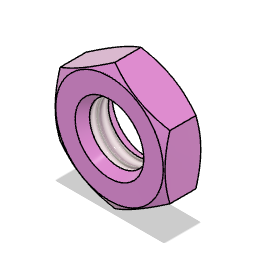
stepper_with_joints v8 (Autodesk Fusion 360 archive; units mm, degrees)
design "Hexagon Thin Nut DIN 439-2 - M5 x 0.8 Steel 6 Plain"
description: Hexagon Thin Nut DIN 439-2 - M5 x 0.8
Autodesk Fusion 360 part; units mm, degrees
note: some values were not read from the file. Chosen so that the rebuilt part matches the saved one: that a step has no effect; which face or edge a step refers to; how an offset face is resized. Set by a fixed rule: which sketch regions a step uses.
sketch "Sketch1" plane through (0, 0, 0) normal (0, 1, 0) x (1, 0, 0)
  line L0 (0, 0) -> (0, -2.7)
  line L1 (-2.5, 0) -> (-3.92, 0)
  line L2 (-3.92, 0) -> (-4.62, -0.4041)
  line L3 (-4.62, -0.4041) -> (-4.62, -2.2959)
  line L4 (-4.62, -2.2959) -> (-3.92, -2.7)
  line L5 (-3.92, -2.7) -> (-2.5, -2.7)
  line L6 (-2.5, -2.7) -> (-2.5, 0)
  dimension "d121" = 5
  dimension "d122" = 30
  dimension "d123" = 30
  dimension "d126" = 2.7
  dimension "d128" = 9.24
  dimension "d172" = 7.84
  constraint vertical L0
  constraint coincident L0 L0.end
  constraint coincident origin L0
  constraint horizontal L1
  constraint perpendicular L1 L3
  constraint perpendicular L3 L5
  constraint perpendicular L5 L6
  constraint coincident L0.start L1
  constraint coincident L0.start origin
  constraint coincident L0.end L5
  constraint equal L1 L5
  measures "d122" angle of L1 L2
  measures "d123" angle of L4 L5
  measures "d126" distance of L1.start L5.end
revolve "Revolve1" add sketch "Sketch1" angle 360 about axis through (0, 0, 0) along (0, 0, 1)
sketch "Sketch8" plane through (0, 0, 2.7) normal (0, 0, 1) x (1, 0, 0)
  line L0 (0, 0) -> (-8, 0) construction
  line L1 (-4, -2.3118) -> (-4, 2.3118)
  circle A0 centre (0, 0) radius 2.5
  circle A1 centre (0, 0) radius 4.62
  dimension "d114" = 4
  constraint horizontal L0
  constraint perpendicular L0 L1
  constraint midpoint L0 L1
  constraint coincident L0.start A0.centre
  constraint coincident L1.end A1
  measures "d114" distance of L0.start L1
extrude "Extrude5" cut sketch "Sketch8" against normal blind 2.7 contours L1 A1 picked at (-4.1, -0.5631)
pattern_circular "C-Pattern2" count 6 over 360 about axis through (0, 0, 1.75) along (0, 0, 1) of "Extrude5"
thread "Thread3" "ISO Metric profile 5.0 M5x0.8 6H" major diameter 5.12 minor diameter 4.234 pitch 0.8 angle 60 resizes the face on face at (-2.4969, 0.1246, 1.8)
sketch "Sketch12" plane through (0, 0, 0) normal (0, 1, 0) x (1, 0, 0)
  line L0 (2.117, -2.7) -> (-2.117, -2.7)
  line L1 (3.92, -2.7) -> (-3.92, -2.7)
  line L2 (3.92, 0) -> (-3.92, 0)
  line L3 (2.117, 0) -> (-2.117, 0)
  line L4 (-2.5, 0) -> (0, 0)
  line L5 (-1.7206, -1.35) -> (-2.5, 0)
  line L6 (-2.5, -2.7) -> (0, -2.7)
  line L7 (-1.7206, -1.35) -> (-2.5, -2.7)
  line L8 (0, 0) -> (0, -2.7)
  dimension "d165" = 60
  dimension "d169" = 60
  dimension "d170" = 2.5
  constraint horizontal L4
  constraint collinear L1 L6
  constraint coincident L5.start L7.start
  constraint vertical L4.start L6.start
  constraint coincident L1 L6.end
  constraint coincident L6.end L8.end
  constraint coincident L4.end L8.start
  measures "d165" angle of L2 L5
  measures "d169" angle of L6 L7
  measures "d170" distance of L4.start L4.end
revolve "Revolve3" cut sketch "Sketch12" angle 360 about axis through (0, 0, 1.75) along (0, 0, 1)
equation "adsk_nheig = 2.70 mm"
equation "adsk_maxdia = 9.24 mm"
equation "adsk_nomdia = 5.00 mm"
equation "d89 = -adsk_nheig"
equation "adsk_waflat = 8.00 mm"
equation "d114 = adsk_waflat / 2"
equation "adsk_chamang1 = 30.00 deg"
equation "adsk_chamang2 = 30.00 deg"
equation "d121 = adsk_nomdia"
equation "d122 = adsk_chamang1"
equation "d123 = adsk_chamang2"
equation "d126 = adsk_nheig"
equation "d128 = adsk_maxdia"
equation "d163 = adsk_nheig"
equation "d170 = adsk_nomdia * 0.5"
equation "adsk_beardia = adsk_waflat * 0.98"
equation "d172 = adsk_beardia"

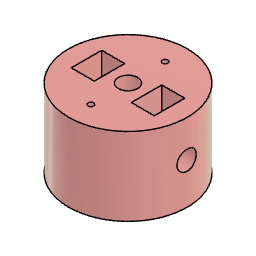
design "nema17 shaft coupler"
Autodesk Fusion 360 part; units mm, degrees
sketch "Sketch1" plane through (0, 0, 0) normal (0, 0, 1) x (1, 0, 0)
  circle A0 centre (0, 0) radius 21
  circle A1 centre (0, 0) radius 2.6
  dimension "d1" = 42
  dimension "d2" = 5.2
  constraint coincident A0.centre A1.centre
  measures "d1" diameter of A0
  measures "d2" diameter of A1
extrude "Extrude1" [suppressed]
sketch "Sketch2" plane through (0, 0, 15) normal (0, 0, 1) x (-1, 0, 0)
  circle A0 centre (0, 0) radius 1.375
  circle A1 centre (0, 0) radius 21
  line L0 (-5, -5.1) -> (-10.2, -5.1)
  line L1 (-10.2, -5.1) -> (-10.2, 5.1)
  line L2 (-10.2, 5.1) -> (-5, 5.1)
  line L3 (-5, 5.1) -> (-5, -5.1)
  line L4 (0, 0) -> (-5, 0)
  dimension "d5" = 5.2
  dimension "d6" = 10.2
  dimension "d7" = 5
  constraint horizontal L0
  constraint vertical L1
  constraint horizontal L2
  constraint vertical L3
  constraint coincident A0.centre A1.centre
  constraint horizontal L4
  constraint midpoint L3 L4.end
  measures "d5" distance of L0.start L0.end
  measures "d6" distance of L0.start L2.end
  measures "d7" distance of A0.centre L4.end
extrude "Extrude2" cut sketch "Sketch2" against normal blind 10 contours L0 L1 L2 L3
ref_plane "WorkPlane1" through (0, 0, 22) normal (0, 0, 1) x (1, 0, 0)
sketch "Sketch3" plane through (5, 0, 0) normal (1, 0, 0) x (0, 1, 0)
  line L0 (5.1, 15) -> (-5.1, 15)
  line L1 (-5.1, 15) -> (-5.1, 5)
  line L2 (-5.1, 5) -> (5.1, 5)
  line L3 (5.1, 5) -> (5.1, 15)
  circle A0 centre (0, 5) radius 3.1
  dimension "d11" = 6.2
  constraint midpoint L2 A0.centre
  measures "d11" diameter of A0
extrude "Extrude3" [no effect]
sketch "Sketch4" plane through (0, 0, 0) normal (0, 0, 1) x (1, 0, 0)
  circle A0 centre (0, 0) radius 16
  circle A1 centre (0, 0) radius 2.6
  dimension "d15" = 32
  dimension "d16" = 5.2
  constraint coincident A0.centre A1.centre
  measures "d15" diameter of A0
  measures "d16" diameter of A1
extrude "Extrude4" add sketch "Sketch4" along normal blind 21 separate body
sketch "Sketch5" plane through (0, 0, 21) normal (0, 0, 1) x (-1, 0, 0)
  circle A0 centre (0, 0) radius 2.6
  circle A1 centre (0, 0) radius 16
  line L0 (-5, -4.1) -> (-11.2, -4.1)
  line L1 (-11.2, -4.1) -> (-11.2, 4.1)
  line L2 (-11.2, 4.1) -> (-5, 4.1)
  line L3 (-5, 4.1) -> (-5, -4.1)
  line L4 (0, 0) -> (-5, 0) construction
  dimension "d19" = 6.2
  dimension "d20" = 8.2
  dimension "d21" = 5
  constraint horizontal L0
  constraint vertical L1
  constraint horizontal L2
  constraint vertical L3
  constraint coincident A0.centre A1.centre
  constraint horizontal L4
  constraint midpoint L3 L4.end
  measures "d19" distance of L0.start L0.end
  measures "d20" distance of L0.start L2.end
  measures "d21" distance of A0.centre L4.end
extrude "Extrude5" cut sketch "Sketch5" against normal blind 10 contours L0 L1 L2 L3
sketch "Sketch6" plane through (5, 0, 0) normal (1, 0, 0) x (0, 1, 0)
  line L0 (4.1, 21) -> (-4.1, 21)
  line L1 (-4.1, 21) -> (-4.1, 11)
  line L2 (-4.1, 11) -> (4.1, 11)
  line L3 (4.1, 11) -> (4.1, 21)
  circle A0 centre (0, 11) radius 2.6
  dimension "d24" = 5.2
  constraint midpoint L2 A0.centre
  measures "d24" diameter of A0
extrude "Extrude6" cut sketch "Sketch6" along normal through all and the other way blind 5 contours L2 A0 | L2 A0
sketch "Sketch7" plane through (5, 0, 0) normal (1, 0, 0) x (0, 1, 0)
  arc A0 (2.6, 11) -> (-2.6, 11) centre (0, 11) ccw
  line L0 (2.6, 11) -> (4.1, 11)
  line L1 (4.1, 11) -> (4.1, 21)
  line L2 (4.1, 21) -> (-4.1, 21)
  line L3 (-4.1, 21) -> (-4.1, 11)
  line L4 (-4.1, 11) -> (-2.6, 11)
  line L5 (4.1, 13.3671) -> (0, 15.7343)
  line L6 (0, 15.7343) -> (-4.1, 13.3671)
  line L7 (-4.1, 13.3671) -> (-4.1, 8.6329)
  line L8 (-4.1, 8.6329) -> (0, 6.2657)
  line L9 (0, 6.2657) -> (4.1, 8.6329)
  line L10 (4.1, 8.6329) -> (4.1, 13.3671)
  point P0 (0, 11)
  constraint coincident P0 A0.centre
  constraint midpoint L0.end L10
extrude "Extrude7" cut sketch "Sketch7" along normal blind 5.2 contours A0 L0 L4 L7 L8 L9 L10 | A0 L0 L1 L3 L4 L5 L6 L7 L10
sketch "Sketch8" plane through (0, 0, 21) normal (0, 0, 1) x (-1, 0, 0)
  line L0 (-11.2, -4.1) -> (-11.2, 4.1)
  line L1 (-11.2, 4.1) -> (-5, 4.1)
  line L2 (-5, 4.1) -> (-5, -4.1)
  line L3 (-5, -4.1) -> (-11.2, -4.1)
  circle A0 centre (0, 0) radius 2.6
  circle A1 centre (0, 0) radius 16
  circle A2 centre (0, -10) radius 0.75
  line L4 (0, 0) -> (16, 0) construction
  circle A3 centre (0, 10) radius 0.75
  dimension "d30" = 1.5
  dimension "d31" = 10
  constraint coincident A0.centre A1.centre
  constraint coincident A1 L4.end
  constraint horizontal L4
  constraint vertical A0.centre A2.centre
  constraint symmetric A2 L4 A3
  measures "d30" diameter of A2
  measures "d31" vertical distance of A0.centre A2.centre
extrude "Extrude8" cut sketch "Sketch8" against normal blind 6 contours A2 | A3
mirror "Mirror1" about plane through (0, 0, 0) normal (1, 0, 0) of "Extrude5", "Extrude6", "Extrude7"

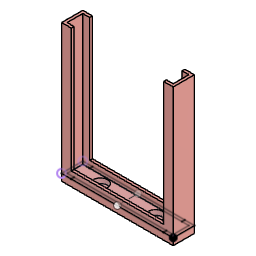
design "pan holder 2"
Autodesk Fusion 360 part; units mm, degrees
sketch "Sketch1" plane through (0, 0, 0) normal (0, 0, 1) x (1, 0, 0)
  line L0 (0, 0) -> (81.3, 0)
  line L1 (81.3, 0) -> (81.3, 15.4)
  line L2 (81.3, 15.4) -> (0, 15.4)
  line L3 (0, 15.4) -> (0, 0)
  dimension "d8" = 81.3
  dimension "d9" = 15.4
  constraint horizontal L0
  constraint vertical L1
  constraint horizontal L2
  constraint vertical L3
  constraint coincident L0.start L3.end
  measures "d8" distance of L0.start L0.end
  measures "d9" distance of L0.start L2.end
extrude "Extrude1" add sketch "Sketch1" along normal blind 5
sketch "Sketch2" plane through (0, 0, 5) normal (0, 0, 1) x (-1, 0, 0)
  line L0 (0, -15.4) -> (0, 0)
  line L1 (0, 0) -> (-81.3, 0)
  line L2 (-81.3, 0) -> (-81.3, -15.4)
  line L3 (-81.3, -15.4) -> (0, -15.4)
  circle A0 centre (-20.65, -7.7) radius 2.6
  circle A1 centre (-20.65, -7.7) radius 5.1
  line L4 (-40.65, -15.4) -> (-40.65, -7.6842) construction
  line L5 (-40.65, -7.7) -> (-81.3, -7.7) construction
  circle A2 centre (-60.65, -7.7) radius 5.1
  circle A3 centre (-60.65, -7.7) radius 2.6
  dimension "d16" = 5.2
  dimension "d18" = 7.7
  dimension "d19" = 10.2
  dimension "d34" = 20
  constraint midpoint L3 L4.start
  constraint midpoint L2 L5.end
  constraint horizontal L5
  constraint vertical L4
  constraint coincident A0.centre L5
  constraint coincident A0.centre A1.centre
  constraint symmetric A0 L4 A3
  constraint symmetric A1 L4 A2
  measures "d16" diameter of A0
  measures "d18" distance of L3 A0.centre
  measures "d19" diameter of A1
  measures "d34" distance of A0.centre L4
extrude "Extrude2" cut sketch "Sketch2" against normal blind 5 contours A0 | A3
extrude "Extrude3" cut sketch "Sketch2" against normal blind 3.6 contours A1 | A2
sketch "Sketch3" plane through (0, 0, 5) normal (0, 0, 1) x (1, 0, 0)
  line L0 (40.65, 14.9854) -> (40.65, -0.0146) construction
  line L1 (0, 15.4) -> (0, 0) construction
  line L2 (74.3, 15.4) -> (74.3, 13.4)
  line L3 (74.3, 13.4) -> (79.3, 13.4)
  line L4 (79.3, 13.4) -> (79.3, 2)
  line L5 (79.3, 2) -> (74.3, 2)
  line L6 (74.3, 2) -> (74.3, 0)
  line L7 (74.3, 0) -> (81.3, 0)
  line L8 (81.3, 0) -> (81.3, 15.4)
  line L9 (81.3, 15.4) -> (74.3, 15.4)
  line L10 (0, 0) -> (0, 15.4)
  line L11 (2, 13.4) -> (2, 2)
  line L12 (2, 2) -> (7, 2)
  line L13 (7, 13.4) -> (2, 13.4)
  line L14 (7, 0) -> (0, 0)
  line L15 (7, 15.4) -> (7, 13.4)
  line L16 (0, 15.4) -> (7, 15.4)
  line L17 (7, 2) -> (7, 0)
  line L18 (7, 15.4) -> (74.3, 15.4)
  line L19 (74.3, 15.4) -> (74.3, 13.4)
  line L20 (74.3, 13.4) -> (7, 13.4)
  line L21 (7, 13.4) -> (7, 15.4)
  line L22 (74.3, 2) -> (7, 2)
  line L23 (7, 2) -> (7, 0)
  line L24 (7, 0) -> (74.3, 0)
  line L25 (74.3, 0) -> (74.3, 2)
  point P0 (81.3, 0)
  dimension "d24" = 40.65
  dimension "d25" = 2
  dimension "d26" = 15.4
  dimension "d27" = 2
  dimension "d29" = 5
  constraint vertical L0
  constraint vertical L2
  constraint perpendicular L2 L3
  constraint perpendicular L3 L4
  constraint perpendicular L2 L5
  constraint perpendicular L5 L6
  constraint perpendicular L6 L7
  constraint perpendicular L5 L8
  constraint perpendicular L2 L9
  constraint equal L2 L6
  constraint equal L3 L5
  constraint symmetric L0 L2.start L15.start
  constraint symmetric L0 L2.end L13.start
  constraint symmetric L0 L3.end L11.start
  constraint symmetric L0 L4.end L11.end
  constraint symmetric L0 L5.end L12.end
  constraint symmetric L0 L6.end L14.start
  constraint symmetric L0 P0 L1.end
  constraint symmetric L0 L8.end L1.start
  constraint coincident P0 L7.end
  constraint horizontal L18
  constraint vertical L19
  constraint horizontal L20
  constraint vertical L21
  constraint horizontal L22
  constraint vertical L23
  constraint horizontal L24
  constraint vertical L25
  measures "d24" distance of L0 L1
  measures "d25" distance of L2.start L2.end
  measures "d26" distance of P0 L8.end
  measures "d27" distance of L4 L8
  measures "d29" distance of L2.end L3.end
extrude "Extrude4" add sketch "Sketch3" along normal blind 95.16 contours L2 L3 L4 L5 L6 L7 L8 L9 L19 L25 | L10 L11 L12 L13 L14 L15 L16 L17 L21 L23
extrude "Extrude5" add sketch "Sketch3" along normal blind 5 contours L2 L15 L18 L19 L20 L21 | L6 L17 L22 L23 L24 L25
equation "pw = 74.8 mm"
equation "pd = 8.9 mm"
equation "ph = 158.6 mm"
equation "clearance = 1.25 mm"
equation "wall_thick = 2 mm"
equation "outer_w = 2 * clearance + 2 * wall_thick + pw"
equation "outer_d = 2 * clearance + 2 * wall_thick + pd"
equation "d8 = outer_w"
equation "d9 = outer_d"
equation "d18 = outer_d / 2"
equation "d24 = outer_w / 2"
equation "d25 = wall_thick"
equation "d26 = outer_d"
equation "d27 = wall_thick"
equation "d30 = ph * 0.6"

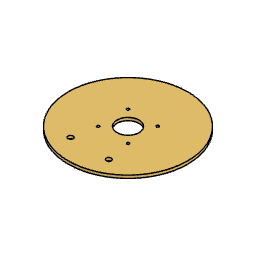
design "top mounting plate"
Autodesk Fusion 360 part; units mm, degrees
sketch "Sketch1" plane through (0, 0, 0) normal (0, 0, 1) x (1, 0, 0)
  circle A0 centre (0, 0) radius 62.5
  line L0 (-16.9429, 20.65) -> (-20.65, 16.9429)
  line L1 (-20.65, -16.9429) -> (-16.9429, -20.65)
  line L2 (-16.9429, -20.65) -> (16.9429, -20.65)
  line L3 (16.9429, 20.65) -> (-16.9429, 20.65)
  line L4 (-20.65, 16.9429) -> (-20.65, -16.9429)
  line L5 (20.65, 16.9429) -> (16.9429, 20.65)
  line L6 (16.9429, -20.65) -> (20.65, -16.9429)
  line L7 (20.65, -16.9429) -> (20.65, 16.9429)
  circle A1 centre (0, 0) radius 11.5
  circle A2 centre (-15.5, 15.5) radius 1.35
  circle A3 centre (0, 0) radius 2
  circle A4 centre (0, 0) radius 20.65 construction
  line L8 (0, 0) -> (0, 20.65) construction
  line L9 (0, 0) -> (20.65, 0) construction
  circle A5 centre (15.5, 15.5) radius 1.35
  circle A6 centre (-15.5, -15.5) radius 1.35
  circle A7 centre (15.5, -15.5) radius 1.35
  circle A8 centre (-20, -40) radius 2.6
  circle A9 centre (20, -40) radius 2.6
  dimension "d1" = 125
  dimension "d2" = 23
  dimension "d3" = 2.7
  dimension "d4" = 15.5
  dimension "d5" = 15.5
  dimension "d8" = 5.2
  dimension "d9" = 40
  dimension "d10" = 20
  constraint coincident A0.centre A1.centre
  constraint midpoint L3 L8.end
  constraint midpoint L7 L9.end
  constraint symmetric A2 L8 A5
  constraint symmetric A2 L9 A6
  constraint symmetric L9 A5 A7
  constraint horizontal L9
  constraint vertical L8
  constraint symmetric L8 A8 A9
  measures "d1" diameter of A0
  measures "d2" diameter of A1
  measures "d3" diameter of A2
  measures "d4" vertical distance of A0.centre A2.centre
  measures "d5" horizontal distance of A0.centre A2.centre
  measures "d8" diameter of A8
  measures "d9" distance of L9 A8.centre
  measures "d10" distance of L8 A8.centre
extrude "Extrude1" add sketch "Sketch1" along normal blind 3 contours A0 | L0 L1 L2 L3 L4 L5 L6 L7

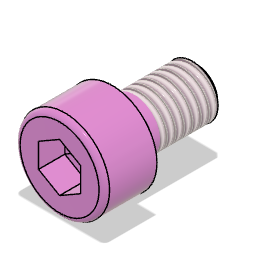
design "Broached Hexagon Socket Head Cap Screw ANSI B18.3.1M - M5x0.8 x 8 Steel Grade 2 Plain"
description: Broached Hexagon Socket Head Cap Screw ANSI B18.3.1M - M5x0.8 x 8
Autodesk Fusion 360 part; units mm, degrees
sketch "Sketch1" plane through (0, 0, 0) normal (0, 1, 0) x (1, 0, 0)
  line L0 (-2.5, 0) -> (-2.5, 8)
  line L1 (-2.5, 8) -> (0, 8)
  line L2 (0, 8) -> (0, -5)
  line L3 (-2.5, 0) -> (-4.25, 0)
  line L4 (-4.25, 0) -> (-4.25, -5)
  line L5 (-4.25, -5) -> (0, -5)
  dimension "d9" = 5
  dimension "d66" = 8.5
  dimension "d68" = 8
  dimension "d79" = 5
  constraint perpendicular L0 L1
  constraint collinear origin L1.end L2.end
  constraint perpendicular L0 L3
  constraint coincident origin L3
  constraint vertical L0
  constraint vertical L2
  constraint parallel L2 L4
  constraint coincident L2 L5.end
  constraint perpendicular L2 L5
  measures "d68" distance of origin L1.end
  measures "d79" distance of L3.end L4.end
revolve "Revolve1" add sketch "Sketch1" angle 360 about axis through (0, 0, -8) along (0, 0, 1)
ref_plane "WorkPlane1" through (0, 0, 5) normal (0, 0, 1) x (1, 0, 0)
sketch "Sketch6" plane through (0, 0, 5) normal (0, 0, 1) x (1, 0, 0)
  line L0 (-2, 0) -> (2, 0) construction
  line L1 (0, 0) -> (-2, 1.1547)
  line L2 (-2, -1.1547) -> (-2, 1.1547)
  line L3 (-2, -1.1547) -> (0, 0)
  dimension "d72" = 4
  dimension "d100" = 150
  constraint horizontal L0
  constraint midpoint L1.start L0
  constraint coincident L1.start L3.end
  constraint perpendicular L0 L2
  constraint midpoint L0.start L2
  constraint coincident L1.end L2.end
  measures "d72" distance of L0.start L0.end
  measures "d100" angle of L0 L1
extrude "Extrude1" cut sketch "Sketch6" against normal blind 2.5
pattern_circular "C-Pattern1" count 6 over 360 about axis through (0, 0, 1.75) along (0, 0, 1) of "Extrude1"
extrude "Extrude2" cut 1 faces at (-0.6667, 0.3849, 2.5) along direction (0, 0, -1) blind 2.5 draft -85
thread "Thread2" "ANSI Metric M Profile 5.0 M5x0.8 4g6g" major diameter 4.901 minor diameter 4.007 pitch 0.8 angle 60 resizes the face on face at (-2.4876, 0.2489, -5.3333)
fillet "Fillet4" radius 0.5 1 edges at (-3.9624, 1.5369, 5)
sketch "Sketch7" plane through (0, 0, 0) normal (0, 1, 0) x (1, 0, 0)
  line L0 (-2.55, 8) -> (-2.55, 7.5092)
  line L1 (-2.55, 7.5092) -> (-2.0092, 8)
  line L2 (0, 8) -> (0, -5)
  line L3 (-2.55, 8) -> (0, 8)
  dimension "d92" = 0.4908
  dimension "d98" = 2.0092
  dimension "d99" = 2.55
  constraint coincident L2.start L3.end
  constraint perpendicular L2 L3
  constraint coincident L1.end L3
  constraint perpendicular L0 L3
  measures "d92" vertical distance of L0.end L1.end
  measures "d98" horizontal distance of origin L1.end
  measures "d99" distance of origin L0
revolve "Revolve3" cut sketch "Sketch7" angle 360 about axis through (0, 0, 1.75) along (0, 0, 1)
equation "d9 = adsk_nomdia"
equation "adsk_nomlen = 8.00 mm"
equation "adsk_headh = 5.00 mm"
equation "adsk_headdia = 8.50 mm"
equation "adsk_nomdia = 5.00 mm"
equation "adsk_philwidth = 4.00 mm"
equation "d31 = -adsk_phildepth"
equation "adsk_phildepth = 2.50 mm"
equation "d66 = adsk_headdia"
equation "d68 = adsk_nomlen"
equation "d71 = adsk_headh"
equation "d72 = adsk_philwidth"
equation "d76 = -adsk_phildepth"
equation "d79 = adsk_headh"
equation "adsk_thrlen = 5.90924 mm"
equation "d84 = adsk_thrlen"
equation "d86 = adsk_nomdia * 0.1"
equation "d92 = adsk_startlen"
equation "adsk_startlen = 0.49076 mm"
equation "adsk_endpointdia = 4.01848 mm"
equation "d98 = adsk_endpointdia / 2"
equation "d99 = adsk_nomdia * 0.51"

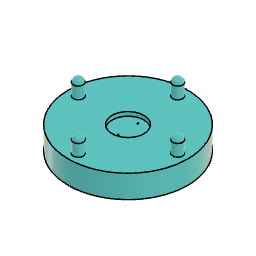
design "nema_bottom_mount"
Autodesk Fusion 360 part; units mm, degrees
sketch "Sketch1" plane through (0, 0, 0) normal (0, 0, 1) x (1, 0, 0)
  circle A0 centre (0, 0) radius 60
  circle A1 centre (0, 0) radius 58.5
  dimension "d1" = 120
  dimension "d2" = 117
  constraint coincident A0.centre A1.centre
  constraint concentric A0 A1
  measures "d1" diameter of A0
  measures "d2" diameter of A1
extrude "Extrude1" add sketch "Sketch1" along normal blind 20
sketch "Sketch2" plane through (0, 0, 20) normal (0, 0, 1) x (-1, 0, 0)
  circle A0 centre (0, 0) radius 58.5
  circle A1 centre (0, 0) radius 60
  circle A2 centre (0, 0) radius 19.2
  dimension "d5" = 38.4
  constraint coincident A0.centre A1.centre
  measures "d5" diameter of A2
extrude "Extrude2" add sketch "Sketch2" along normal blind 3 contours A0 | A1
sketch "Sketch3" plane through (0, 0, 23) normal (0, 0, 1) x (-1, 0, 0)
  circle A0 centre (0, 0) radius 19.2
  circle A1 centre (0, 0) radius 60
  circle A2 centre (0, 0) radius 16
  dimension "d8" = 32
  constraint coincident A0.centre A1.centre
  measures "d8" diameter of A2
extrude "Extrude3" add sketch "Sketch3" against normal blind 4 contours A0
sketch "Sketch4" plane through (0, 0, 19) normal (0, 0, -1) x (1, 0, 0)
  circle A0 centre (0, 0) radius 16
  circle A1 centre (0, 0) radius 19.2
  circle A2 centre (0, 0) radius 19
  circle A3 centre (0, 10) radius 0.75
  line L0 (0, 0) -> (-16, 0) construction
  circle A4 centre (0, -10) radius 0.75
  dimension "d13" = 1.5
  dimension "d14" = 10
  constraint coincident A0.centre A1.centre
  constraint coincident A0 L0.end
  constraint horizontal L0
  constraint vertical A0.centre A3.centre
  constraint symmetric A3 L0 A4
  measures "d13" diameter of A3
  measures "d14" distance of A3.centre L0
extrude "Extrude4" add sketch "Sketch4" along normal blind 3 contours A0 | A1 | A2
sketch "Sketch5" plane through (0, 0, 23) normal (0, 0, 1) x (-1, 0, 0)
  circle A0 centre (0, 0) radius 16
  circle A1 centre (0, 0) radius 60
  circle A2 centre (-50, 0) radius 5
  dimension "d15" = 10
  dimension "d16" = 50
  constraint horizontal A0.centre A2.centre
  measures "d15" diameter of A2
  measures "d16" distance of A0.centre A2.centre
extrude "Extrude5" add sketch "Sketch5" along normal blind 17 contours A2
fillet "Fillet1" radius 5 1 edges at (54.6616, 1.8081, 40)
pattern_circular "C-Pattern1" count 4 over 360 about axis through (0, 0, 23) along (0, 0, -1) of "Extrude5", "Fillet1"
equation "d5 = 32 mm + ( ( 2 * 3 ) * 1 ) * 1 mm + 0.4 mm"
equation "d9 = -5.5 mm + 1.5 mm"
equation "d17 = 24 mm - 5.5 mm - 3 mm + 1.5 mm"

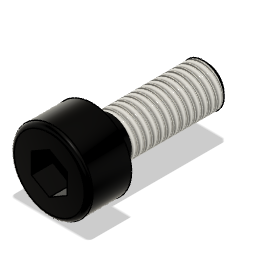
design "Broached Hexagon Socket Head Cap Screw ANSI B18.3.1M - M3x0.5 x 8 Steel Grade 2 Black"
description: Broached Hexagon Socket Head Cap Screw ANSI B18.3.1M - M3x0.5 x 8
Autodesk Fusion 360 part; units mm, degrees
sketch "Sketch1" plane through (0, 0, 0) normal (0, 1, 0) x (1, 0, 0)
  line L0 (-1.5, 0) -> (-1.5, 8)
  line L1 (-1.5, 8) -> (0, 8)
  line L2 (0, 8) -> (0, -3)
  line L3 (-1.5, 0) -> (-2.75, 0)
  line L4 (-2.75, 0) -> (-2.75, -3)
  line L5 (-2.75, -3) -> (0, -3)
  dimension "d9" = 3
  dimension "d66" = 5.5
  dimension "d68" = 8
  dimension "d79" = 3
  constraint perpendicular L0 L1
  constraint collinear origin L1.end L2.end
  constraint perpendicular L0 L3
  constraint coincident origin L3
  constraint vertical L0
  constraint vertical L2
  constraint parallel L2 L4
  constraint coincident L2 L5.end
  constraint perpendicular L2 L5
  measures "d68" distance of origin L1.end
  measures "d79" distance of L3.end L4.end
revolve "Revolve1" add sketch "Sketch1" angle 360 about axis through (0, 0, -8) along (0, 0, 1)
ref_plane "WorkPlane1" through (0, 0, 3) normal (0, 0, 1) x (1, 0, 0)
sketch "Sketch6" plane through (0, 0, 3) normal (0, 0, 1) x (1, 0, 0)
  line L0 (-1.25, 0) -> (1.25, 0) construction
  line L1 (0, 0) -> (-1.25, 0.7217)
  line L2 (-1.25, -0.7217) -> (-1.25, 0.7217)
  line L3 (-1.25, -0.7217) -> (0, 0)
  dimension "d72" = 2.5
  dimension "d100" = 150
  constraint horizontal L0
  constraint midpoint L1.start L0
  constraint coincident L1.start L3.end
  constraint perpendicular L0 L2
  constraint midpoint L0.start L2
  constraint coincident L1.end L2.end
  measures "d72" distance of L0.start L0.end
  measures "d100" angle of L0 L1
extrude "Extrude1" cut sketch "Sketch6" against normal blind 1.5
pattern_circular "C-Pattern1" count 6 over 360 about axis through (0, 0, 1.75) along (0, 0, 1) of "Extrude1"
extrude "Extrude2" cut 1 faces at (0, 0.4811, 1.5) along direction (0, 0, -1) blind 1.5 draft -85
thread "Thread2" "ANSI Metric M Profile 3.0 M3x0.5 4g6g" major diameter 2.927 minor diameter 2.369 pitch 0.5 angle 60 resizes the face on face at (-1.4925, 0.1494, -5.3333)
fillet "Fillet4" radius 0.3 1 edges at (-2.5639, 0.9944, 3)
sketch "Sketch7" plane through (0, 0, 0) normal (0, 1, 0) x (1, 0, 0)
  line L0 (-1.53, 8) -> (-1.53, 7.6933)
  line L1 (-1.53, 7.6933) -> (-1.1933, 8)
  line L2 (0, 8) -> (0, -3)
  line L3 (-1.53, 8) -> (0, 8)
  dimension "d92" = 0.3067
  dimension "d98" = 1.1933
  dimension "d99" = 1.53
  constraint coincident L2.start L3.end
  constraint perpendicular L2 L3
  constraint coincident L1.end L3
  constraint perpendicular L0 L3
  measures "d92" vertical distance of L0.end L1.end
  measures "d98" horizontal distance of origin L1.end
  measures "d99" distance of origin L0
revolve "Revolve3" cut sketch "Sketch7" angle 360 about axis through (0, 0, 1.75) along (0, 0, 1)
equation "d9 = adsk_nomdia"
equation "adsk_nomlen = 8.00 mm"
equation "adsk_headh = 3.00 mm"
equation "adsk_headdia = 5.50 mm"
equation "adsk_nomdia = 3.00 mm"
equation "adsk_philwidth = 2.50 mm"
equation "d31 = -adsk_phildepth"
equation "adsk_phildepth = 1.50 mm"
equation "d66 = adsk_headdia"
equation "d68 = adsk_nomlen"
equation "d71 = adsk_headh"
equation "d72 = adsk_philwidth"
equation "d76 = -adsk_phildepth"
equation "d79 = adsk_headh"
equation "adsk_thrlen = 6.693275 mm"
equation "d84 = adsk_thrlen"
equation "d86 = adsk_nomdia * 0.1"
equation "d92 = adsk_startlen"
equation "adsk_startlen = 0.306725 mm"
equation "adsk_endpointdia = 2.38655 mm"
equation "d98 = adsk_endpointdia / 2"
equation "d99 = adsk_nomdia * 0.51"
